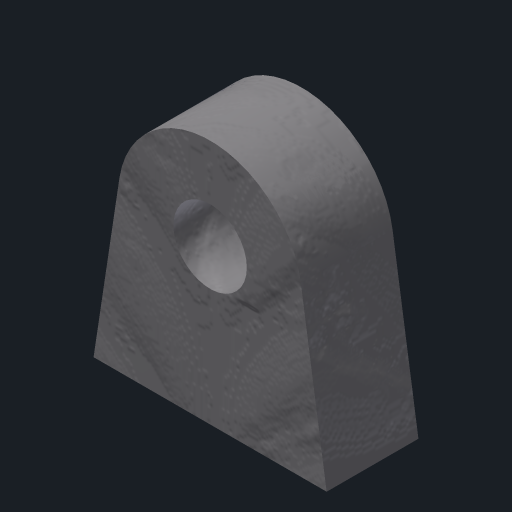
# Autodesk Inventor part: OTRO_EXTREMO
Saved by Autodesk Inventor 2024.3 (Build 283343000, 343)
## iProperties
Created: 2024-08-24
Part Number: OTRO_EXTREMO
Material: Steel, Mild, Welded
Document SubType Name: Modeling
Designer: Niler
Density: 7.85 g/cm^3
Appearance: Weld - Steel Mild
Author: Niler
Autodesk Inventor part; units mm, degrees
ref_plane "YZ Plane" through (0, 0, 0) normal (1, 0, 0) x (0, 1, 0)
ref_plane "XZ Plane" through (0, 0, 0) normal (0, 1, 0) x (-1, 0, 0)
ref_plane "XY Plane" through (0, 0, 0) normal (0, 0, 1) x (1, 0, 0)
sketch "Sketch1" plane through (0, 0, 0) normal (0, 0, 1) x (1, 0, 0)
  circle A0 centre (0, 16.7917) radius 4
  circle A1 centre (0, 16.7917) radius 10
  line L0 (-9.8838, 18.3117) -> (-12.7, 0)
  line L1 (-12.7, 0) -> (0, 0)
  line L2 (0, 0) -> (0, 16.7917)
  line L3 (9.8838, 18.3117) -> (12.7, 0)
  line L4 (12.7, 0) -> (0, 0)
  dimension "d1" = 20
  dimension "d0" = 8
  dimension "d2" = 25.4
  constraints: 10 end point, 2 symmetric about line, 1 centre point, 1 coincident, 1 horizontal, 1 perpendicular, 4 other
  measures "d0" diameter of A0
  measures "d2" distance of L3.end L0.end
extrude "Extrusion1" add sketch "Sketch1" along normal blind 10
body "Solid1"
